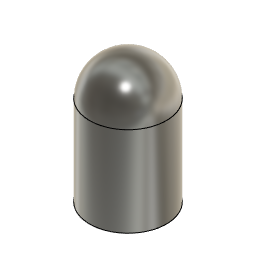
life v2 (Autodesk Fusion 360 design; units mm, degrees)
Autodesk Fusion 360 part; units mm, degrees
sketch "Esquisse1" plane through (0, 0, 0) normal (0, 0, 1) x (1, 0, 0)
  circle A0 centre (0, 0) radius 15
  dimension "d1" = 30
  constraint coincident A0.centre origin
  measures "d1" diameter of A0
extrude "Extrusion1" add sketch "Esquisse1" along normal blind 50
fillet "Congé1" radius 15 1 faces at (3.6653, 3.4009, 50)
sketch "Esquisse2" plane through (0, 0, 0) normal (0, 0, 1) x (1, 0, 0)
  circle A0 centre (0, 0) radius 5
  dimension "d6" = 10
  constraint coincident A0.centre origin
  measures "d6" diameter of A0
extrude "Extrusion2" cut sketch "Esquisse2" along normal blind 2.5
